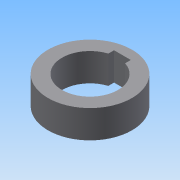
# Autodesk Inventor part: 中间传动大锥齿轮
Saved by Autodesk Inventor 2015 (Build 190159000, 159)
## iProperties
Created: 2017-05-27
Part Number: 中间传动大锥齿轮
Material: 常规
Document SubType Name: Modeling
Designer: Administrator
Density: 1 g/cm^3
Appearance: 默认
Author: Administrator
Autodesk Inventor part; units mm, degrees
ref_plane "YZ Plane" through (0, 0, 0) normal (1, 0, 0) x (0, 1, 0)
ref_plane "XZ Plane" through (0, 0, 0) normal (0, 1, 0) x (-1, 0, 0)
ref_plane "XY Plane" through (0, 0, 0) normal (0, 0, 1) x (1, 0, 0)
sketch "草图1" plane through (0, 0, 0) normal (0, 0, 1) x (1, 0, 0)
  circle A0 centre (0, 0) radius 15
  circle A1 centre (0, 0) radius 10
  dimension "d0" = 30
  dimension "d1" = 20
  constraints: 2 centre point, 2 coincident
  measures "d0" diameter of A0
  measures "d1" diameter of A1
extrude "拉伸1" add sketch "草图1" along normal blind 10
sketch "草图2" plane through (0, 0, 10) normal (0, 0, 1) x (1, 0, 0)
  line L0 (-3, 11.6) -> (3, 11.6)
  line L1 (3, 11.6) -> (3, 10)
  line L2 (3, 10) -> (-3, 10)
  line L3 (-3, 10) -> (-3, 11.6)
  circle A0 centre (0, 0) radius 10 projected
  line L4 (-3, 10) -> (-3, 9.5394)
  line L5 (3, 10) -> (3, 9.5394)
  circle A1 centre (0, 0) radius 10 projected
  arc A2 (3, 9.5394) -> (-3, 9.5394) centre (0, 0) ccw
  point P0 (0, 10)
  dimension "d4" = 6
  dimension "d5" = 1.6
  constraints: 12 end point, 5 point on circle, 2 parallel, 1 centre point, 1 collinear, 1 concentric, 1 horizontal, 1 midpoint, 1 perpendicular, 1 tangent, 1 vertical, 2 other
  measures "d4" distance of L1.end L2.end
  measures "d5" distance of L0.end L1.end
extrude "拉伸2" cut sketch "草图2" against normal blind 10 contours L0 L1 L2 L3 | L2 A0 L4 | L5 A0 L2
